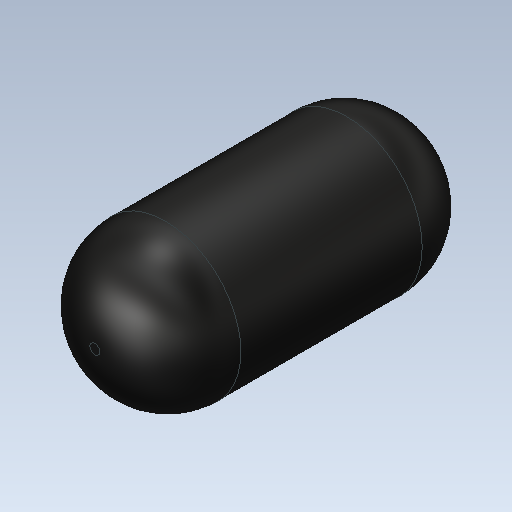
# Autodesk Inventor part: actuator_counterweight
Saved by Autodesk Inventor 2020 (Build 240168000, 168)
## iProperties
Created: 2017-12-01
Part Number: actuator_counterweight
Material: Lead
Document SubType Name: Modeling
Designer: stedrock
Density: 11.34 g/cm^3
Appearance: Lead
Mass: 55.2305 g
Surface Area: 15.3464 cm^2
Volume: 4.87042 cm^3
Author: stedrock
Autodesk Inventor part; units mm, degrees
ref_plane "YZ Plane" through (0, 0, 0) normal (1, 0, 0) x (0, 1, 0)
ref_plane "XZ Plane" through (0, 0, 0) normal (0, 1, 0) x (-1, 0, 0)
ref_plane "XY Plane" through (0, 0, 0) normal (0, 0, 1) x (1, 0, 0)
sketch "Sketch1" plane through (0, 0, 0) normal (0, 0, 1) x (1, 0, 0)
  circle A0 centre (0, 0) radius 7.5
  dimension "d0" = 15
  constraints: 1 centre point, 1 coincident
  measures "d0" diameter of A0
extrude "Extrusion3" add sketch "Sketch1" along normal blind 32
fillet "Fillet2" radius 7 2 edges at (-7.5, 0, 32) (-7.5, 0, 0)
body "Solid2"
